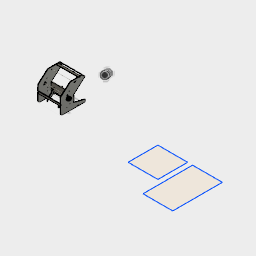
karaoke (Autodesk Fusion 360 design; units mm, degrees)
Autodesk Fusion 360 part; units mm, degrees
(part 1 of 3)
sketch "karaoke_machine_CNC" plane through (0, 0, 0) normal (1, 0, 0) x (0, 0, -1)
  line L0 (-550.0191, 0.004) -> (-575.0344, 25.0175)
  line L1 (-565.5925, 332.4848) -> (-375.0549, 500.0614)
  circle A0 centre (-278.825, 453.825) radius 8.595
  circle A1 centre (-294.0872, 469.0872) radius 1.445
  circle A2 centre (-263.5628, 469.0872) radius 1.445
  circle A3 centre (-294.0872, 438.5628) radius 1.445
  circle A4 centre (-263.5628, 438.5628) radius 1.445
  circle A5 centre (-400, 350) radius 4
  circle A6 centre (-300.125, 453.825) radius 7.88
  circle A7 centre (-380, 180) radius 4
  circle A8 centre (-450, 90) radius 4
  circle A9 centre (-385, 120) radius 4
  circle A10 centre (43.7005, 245.2652) radius 4
  spline S0 degree 5 poles (123.7005, 365.2652) (122.0522, 364.7199) (118.9216, 363.5317) (114.724, 361.457) (110.1257, 358.1046) (106.0037, 352.9433) (103.3614, 346.847) (101.891, 339.898) (101.0418, 332.2492) (100.1108, 324.1052) (98.3724, 315.6927) (95.1998, 307.2345) (90.1793, 298.924) (83.2582, 290.8942) (74.6972, 283.2208) (64.9664, 275.9336) (54.6633, 269.0254) (44.4241, 262.4607) (34.8373, 256.1846) (26.3611, 250.1305) (19.2237, 244.2286) (13.4655, 238.4105) (9.0045, 232.6126) (5.6928, 226.78) (3.3728, 220.8704) (1.9392, 214.8586) (1.457, 209.9581) (1.4586, 206.23) (1.6207, 203.7212) (1.742, 202.461) knots 0 0 0 0 0 0 0.04 0.08 0.12 0.16 0.2 0.24 0.28 0.32 0.36 0.4 0.44 0.48 0.52 0.56 0.6 0.64 0.68 0.72 0.76 0.8 0.84 0.88 0.92 0.96 1 1 1 1 1 1
  line L2 (123.7005, 365.2652) -> (143.7005, 365.2652)
  circle A11 centre (108.7005, 275.2652) radius 4
  circle A12 centre (113.7005, 335.2652) radius 4
  spline S1 degree 5 poles (143.7005, 365.2652) (142.5207, 363.6794) (140.2638, 360.5375) (137.1859, 355.9139) (133.6982, 349.93) (130.3733, 342.6612) (128.0779, 335.363) (126.8118, 327.4866) (126.5171, 318.2243) (126.7275, 307.7361) (126.8179, 296.5667) (126.1032, 285.5142) (123.9849, 275.3406) (120.1067, 266.502) (114.4031, 259.0526) (107.008, 252.8039) (98.2027, 247.4139) (88.3531, 242.4959) (77.8463, 237.7348) (67.0572, 232.924) (56.3415, 227.9315) (46.021, 222.6873) (36.3716, 217.1625) (27.6109, 211.3538) (19.8803, 205.2637) (13.2549, 198.8948) (8.8635, 193.5794) (6.083, 189.4699) (4.4567, 186.6759) (3.7005, 185.2652) knots 0 0 0 0 0 0 0.04 0.08 0.12 0.16 0.2 0.24 0.28 0.32 0.36 0.4 0.44 0.48 0.52 0.56 0.6 0.64 0.68 0.72 0.76 0.8 0.84 0.88 0.92 0.96 1 1 1 1 1 1
  line L3 (131.9605, 355.3516) -> (123.6339, 309.9117)
  line L4 (1.742, 202.461) -> (3.7005, 185.2652)
  circle A13 centre (-26.463, 282.4606) radius 4
  line L5 (53.537, 402.4606) -> (73.537, 402.4606)
  line L6 (-68.4215, 239.6564) -> (-66.463, 222.4606)
  spline S2 degree 5 poles (73.537, 402.4606) (72.3573, 400.8748) (70.1003, 397.7329) (67.0225, 393.1093) (63.5347, 387.1254) (60.2099, 379.8566) (57.9144, 372.5584) (56.6484, 364.682) (56.3536, 355.4197) (56.564, 344.9315) (56.6544, 333.7621) (55.9397, 322.7096) (53.8214, 312.536) (49.9432, 303.6974) (44.2396, 296.248) (36.8445, 289.9993) (28.0392, 284.6094) (18.1896, 279.6913) (7.6828, 274.9302) (-3.1063, 270.1194) (-13.822, 265.127) (-24.1425, 259.8827) (-33.7919, 254.3579) (-42.5526, 248.5492) (-50.2832, 242.4591) (-56.9086, 236.0902) (-61.3, 230.7748) (-64.0805, 226.6653) (-65.7068, 223.8713) (-66.463, 222.4606) knots 0 0 0 0 0 0 0.04 0.08 0.12 0.16 0.2 0.24 0.28 0.32 0.36 0.4 0.44 0.48 0.52 0.56 0.6 0.64 0.68 0.72 0.76 0.8 0.84 0.88 0.92 0.96 1 1 1 1 1 1
  line L7 (61.797, 392.547) -> (53.4704, 347.1071)
  circle A14 centre (38.537, 312.4606) radius 4
  circle A15 centre (43.537, 372.4606) radius 4
  spline S3 degree 5 poles (53.537, 402.4606) (51.8887, 401.9153) (48.7582, 400.7271) (44.5605, 398.6524) (39.9622, 395.3) (35.8403, 390.1387) (33.1979, 384.0424) (31.7275, 377.0934) (30.8784, 369.4446) (29.9473, 361.3006) (28.2089, 352.8881) (25.0363, 344.4299) (20.0159, 336.1194) (13.0947, 328.0896) (4.5337, 320.4162) (-5.1971, 313.129) (-15.5002, 306.2208) (-25.7393, 299.6561) (-35.3261, 293.38) (-43.8023, 287.3259) (-50.9398, 281.424) (-56.698, 275.6059) (-61.159, 269.808) (-64.4707, 263.9754) (-66.7907, 258.0658) (-68.2242, 252.054) (-68.7065, 247.1535) (-68.7049, 243.4254) (-68.5428, 240.9166) (-68.4215, 239.6564) knots 0 0 0 0 0 0 0.04 0.08 0.12 0.16 0.2 0.24 0.28 0.32 0.36 0.4 0.44 0.48 0.52 0.56 0.6 0.64 0.68 0.72 0.76 0.8 0.84 0.88 0.92 0.96 1 1 1 1 1 1
  line L8 (-597.7644, -31.7077) -> (-597.7644, -51.7032)
  line L9 (-597.7763, -161.7146) -> (-597.7763, -141.7146)
  line L10 (-312.3162, 219.9099) -> (-312.3331, 234.9601)
  line L11 (-309.8393, 237.6116) -> (-299.7645, 237.6116)
  line L12 (-299.7645, 217.4116) -> (-309.8145, 217.4116)
  arc A16 (-312.3162, 219.9099) -> (-309.8145, 217.4116) centre (-312.3145, 217.4099) ccw
  arc A17 (-309.8393, 237.6116) -> (-312.3331, 234.9601) centre (-312.3347, 237.4601) ccw
  line L13 (-585.2646, -21.7077) -> (-145.2646, -21.7033)
  line L14 (-585.2759, -171.7145) -> (-145.2759, -171.7005)
  line L15 (-142.8943, -31.6974) -> (-132.8943, -31.6974)
  line L16 (-132.8943, -31.6974) -> (-132.8943, -51.7032)
  line L17 (-132.8943, -51.7032) -> (-142.8887, -51.7032)
  line L18 (-133.0064, -161.6675) -> (-133.0064, -141.7032)
  line L19 (-585.253, -29.2077) -> (-585.2646, -21.7077)
  line L20 (-585.3327, -54.2032) -> (-585.3327, -139.2151)
  line L21 (-585.2785, -164.2145) -> (-585.2759, -171.7145)
  line L22 (-145.3891, -54.197) -> (-145.3747, -139.2034)
  line L23 (-145.2785, -164.1551) -> (-145.2759, -171.7005)
  line L24 (-145.2646, -21.7033) -> (-145.2644, -29.2004)
  arc A18 (-145.3946, -34.197) -> (-142.8943, -31.6974) centre (-145.3943, -31.697) ccw
  arc A19 (-145.2644, -29.2004) -> (-145.3946, -34.197) centre (-145.3943, -31.697) ccw
  arc A20 (-145.3883, -49.197) -> (-145.3891, -54.197) centre (-145.3887, -51.697) ccw
  arc A21 (-142.8887, -51.7032) -> (-145.3883, -49.197) centre (-145.3887, -51.697) ccw
  arc A22 (-145.3747, -139.2034) -> (-145.3328, -144.2032) centre (-145.3328, -141.7031) ccw
  arc A23 (-143.0064, -161.6675) -> (-145.5046, -159.1655) centre (-145.5064, -161.6655) ccw
  arc A24 (-145.5046, -159.1655) -> (-145.2785, -164.1551) centre (-145.5064, -161.6655) ccw
  arc A25 (-587.7774, -141.7146) -> (-585.2773, -144.2145) centre (-585.2774, -141.7145) ccw
  arc A26 (-585.2773, -144.2145) -> (-585.3327, -139.2151) centre (-585.2774, -141.7145) ccw
  arc A27 (-585.2764, -159.2145) -> (-587.7763, -161.7146) centre (-585.2763, -161.7145) ccw
  arc A28 (-585.2785, -164.2145) -> (-585.2764, -159.2145) centre (-585.2763, -161.7145) ccw
  arc A29 (-585.3328, -49.2032) -> (-587.8328, -51.7032) centre (-585.3328, -51.7032) ccw
  arc A30 (-585.3327, -54.2032) -> (-585.3328, -49.2032) centre (-585.3328, -51.7032) ccw
  arc A31 (-587.7644, -31.7077) -> (-585.2643, -34.2077) centre (-585.2644, -31.7077) ccw
  arc A32 (-585.2643, -34.2077) -> (-585.253, -29.2077) centre (-585.2644, -31.7077) ccw
  arc A33 (-145.3328, -144.2032) -> (-142.8328, -141.7032) centre (-145.3328, -141.7032) ccw
  line L25 (-133.0064, -141.7032) -> (-142.8328, -141.7032)
  line L26 (-143.0064, -161.6675) -> (-133.0064, -161.6675)
  line L27 (-587.7644, -31.7077) -> (-597.7644, -31.7077)
  line L28 (-597.7644, -51.7032) -> (-587.8328, -51.7032)
  line L29 (-597.7763, -141.7146) -> (-587.7774, -141.7146)
  line L30 (-587.7763, -161.7146) -> (-597.7763, -161.7146)
  line L31 (-575.4928, 198.8808) -> (-575.7799, 309.8801)
  line L32 (-575.0344, 25.0175) -> (-575.493, 178.6808)
  line L33 (-562.9429, 196.3808) -> (-562.9435, 181.3308)
  line L34 (-565.439, 178.6808) -> (-575.493, 178.6808)
  line L35 (-575.4928, 198.8808) -> (-565.4428, 198.8808)
  arc A34 (-562.9429, 196.3808) -> (-565.4428, 198.8808) centre (-562.9428, 198.8808) ccw
  arc A35 (-565.439, 178.6808) -> (-562.9435, 181.3308) centre (-562.9435, 178.8308) ccw
  arc A36 (-182.4468, 487.9507) -> (-179.7968, 490.4462) centre (-179.9468, 487.9507) ccw
  line L36 (-179.7968, 500.0318) -> (-179.7968, 490.4462)
  line L37 (-182.4468, 487.9507) -> (-197.5, 487.9508)
  line L38 (-199.9968, 490.45) -> (-199.9968, 500.0323)
  arc A37 (-199.9968, 490.45) -> (-197.5, 487.9508) centre (-200, 487.95) ccw
  line L39 (-375.0549, 500.0614) -> (-199.9968, 500.0323)
  line L40 (-179.7968, 500.0318) -> (-124.9386, 500.0255)
  line L41 (-607.4311, 2.1633) -> (-627.4311, 2.1468)
  line L42 (-637.4292, 14.6466) -> (-637.4346, 454.6466)
  line L43 (-597.4308, 454.6468) -> (-597.4308, 14.6571)
  line L44 (-607.4355, 467.1466) -> (-627.4355, 467.1622)
  arc A38 (-627.4313, 12.1468) -> (-629.9313, 14.6468) centre (-627.4313, 14.6468) ccw
  line L45 (-629.9313, 14.6468) -> (-637.4292, 14.6466)
  line L46 (-627.4311, 2.1468) -> (-627.4313, 12.1468)
  line L47 (-607.431, 12.1571) -> (-607.4311, 2.1633)
  line L48 (-597.4308, 14.6571) -> (-604.931, 14.6571)
  line L49 (-637.4346, 454.6466) -> (-629.9354, 454.6466)
  line L50 (-627.4355, 467.1622) -> (-627.4354, 457.1467)
  line L51 (-607.4354, 457.1466) -> (-607.4355, 467.1466)
  line L52 (-604.9354, 454.6467) -> (-597.4308, 454.6468)
  arc A39 (-607.4354, 457.1466) -> (-604.9354, 454.6467) centre (-607.4354, 454.6466) ccw
  arc A40 (-629.9354, 454.6466) -> (-627.4354, 457.1467) centre (-627.4354, 454.6467) ccw
  arc A41 (-604.931, 14.6571) -> (-607.431, 12.1571) centre (-607.431, 14.6571) ccw
  arc A42 (-669.7101, -227.9538) -> (-672.2101, -225.4537) centre (-669.7101, -225.4538) ccw
  line L53 (-229.655, -227.9918) -> (-229.655, -235.4805)
  arc A43 (-227.1554, -225.4914) -> (-229.655, -227.9918) centre (-229.6554, -225.4918) ccw
  arc A44 (-229.6531, -202.9918) -> (-227.1528, -205.4915) centre (-229.6528, -205.4918) ccw
  line L54 (-669.7101, -235.4805) -> (-669.7101, -227.9538)
  line L55 (-227.1554, -225.4914) -> (-217.1554, -225.4914)
  arc A45 (-672.1536, -205.4537) -> (-669.6531, -202.9539) centre (-669.6536, -205.4539) ccw
  line L56 (-229.6531, -195.4805) -> (-229.6531, -202.9918)
  line L57 (-217.1554, -205.4915) -> (-227.1528, -205.4915)
  line L58 (-217.1554, -225.4914) -> (-217.1554, -205.4915)
  line L59 (-682.1536, -225.4537) -> (-682.1536, -205.4537)
  line L60 (-669.6531, -202.9539) -> (-669.6531, -195.4805)
  line L61 (-672.2101, -225.4537) -> (-682.1536, -225.4537)
  line L62 (-682.1536, -205.4537) -> (-672.1536, -205.4537)
  line L63 (-229.655, -235.4805) -> (-669.7101, -235.4805)
  line L64 (-669.6531, -195.4805) -> (-229.6531, -195.4805)
  line L65 (-214.0002, 187.7845) -> (-264.0002, 187.7845)
  line L66 (-269.0002, 194.7845) -> (-264.0002, 187.7845)
  line L67 (-264.0002, 237.7845) -> (-269.0002, 237.7845)
  line L68 (-214.0002, 237.7845) -> (-209.0002, 237.7845)
  line L69 (-264.0002, 242.7845) -> (-264.0002, 249.7845)
  line L70 (-269.0002, 237.7845) -> (-269.0002, 194.7845)
  arc A46 (-264.0002, 237.7845) -> (-264.0002, 242.7845) centre (-264.0002, 240.2845) ccw
  line L71 (-209.0002, 237.7845) -> (-209.0002, 194.7845)
  arc A47 (-214.0002, 242.7845) -> (-214.0002, 237.7845) centre (-214.0002, 240.2845) ccw
  line L72 (-209.0002, 194.7845) -> (-214.0002, 187.7845)
  line L73 (-264.0002, 249.7845) -> (-214.0002, 249.7845)
  line L74 (-214.0002, 249.7845) -> (-214.0002, 242.7845)
  circle A48 centre (-239.0002, 214.7845) radius 4
  line L75 (-173.2818, 321.1956) -> (-130.9318, 321.1956)
  line L76 (-130.9318, 321.1956) -> (-130.9318, 278.8456)
  line L77 (-130.9318, 278.8456) -> (-173.2818, 278.8456)
  line L78 (-173.2818, 278.8456) -> (-173.2818, 321.1956)
  arc A49 (-184.0002, 237.7845) -> (-184.0002, 242.7845) centre (-184.0002, 240.2845) ccw
  line L79 (-184.0002, 242.7845) -> (-184.0002, 249.7845)
  arc A50 (-134.0002, 242.7845) -> (-134.0002, 237.7845) centre (-134.0002, 240.2845) ccw
  line L80 (-129.0002, 237.7845) -> (-129.0002, 194.7845)
  line L81 (-134.0002, 237.7845) -> (-129.0002, 237.7845)
  line L82 (-134.0002, 249.7845) -> (-134.0002, 242.7845)
  line L83 (-189.0002, 194.7845) -> (-184.0002, 187.7845)
  line L84 (-184.0002, 237.7845) -> (-189.0002, 237.7845)
  line L85 (-184.0002, 249.7845) -> (-134.0002, 249.7845)
  line L86 (-134.0002, 187.7845) -> (-184.0002, 187.7845)
  line L87 (-189.0002, 237.7845) -> (-189.0002, 194.7845)
  line L88 (-129.0002, 194.7845) -> (-134.0002, 187.7845)
  line L89 (-173.2818, 206.8396) -> (-173.2818, 208.8983)
  line L90 (-183.2818, 326.1956) -> (-178.2818, 331.1956)
  line L91 (-125.9318, 331.1956) -> (-120.9318, 326.1956)
  line L92 (-183.2818, 273.8456) -> (-178.2818, 268.8456)
  line L93 (-125.9318, 268.8456) -> (-120.9318, 273.8456)
  line L94 (-120.9318, 326.1956) -> (-120.9318, 273.8456)
  line L95 (-183.2818, 273.8456) -> (-183.2818, 326.1956)
  line L96 (-125.9318, 268.8456) -> (-178.2818, 268.8456)
  line L97 (-142.1068, 343.1956) -> (-162.1068, 343.1956)
  arc A51 (-164.6068, 331.1956) -> (-162.1068, 333.6956) centre (-162.1068, 331.1956) ccw
  arc A52 (-142.1068, 333.6956) -> (-139.6068, 331.1956) centre (-142.1068, 331.1956) ccw
  line L98 (-142.1068, 333.6956) -> (-142.1068, 343.1956)
  line L99 (-162.1068, 343.1956) -> (-162.1068, 333.6956)
  line L100 (-178.2818, 331.1956) -> (-164.6068, 331.1956)
  line L101 (-139.6068, 331.1956) -> (-125.9318, 331.1956)
  line L102 (-467, 294.9) -> (-466, 294.9)
  line L103 (-438.025, 304.9) -> (-432.025, 304.9)
  line L104 (-428.025, 300.9) -> (-428.025, 283.9)
  line L105 (-432.025, 279.9) -> (-438.025, 279.9)
  line L106 (-442.025, 283.9) -> (-442.025, 300.9)
  arc A53 (-438.025, 304.9) -> (-442.025, 300.9) centre (-438.025, 300.9) ccw
  arc A54 (-428.025, 300.9) -> (-432.025, 304.9) centre (-432.025, 300.9) ccw
  arc A55 (-432.025, 279.9) -> (-428.025, 283.9) centre (-432.025, 283.9) ccw
  arc A56 (-442.025, 283.9) -> (-438.025, 279.9) centre (-438.025, 283.9) ccw
  circle A57 centre (-447.525, 290.8) radius 4
  line L107 (-460.4181, 236.3812) -> (-460.4102, 228.6812)
  line L108 (-457.9075, 226.1839) -> (-412.7075, 226.234)
  line L109 (-410.2102, 228.7367) -> (-410.2169, 236.3845)
  arc A58 (-410.2169, 236.3845) -> (-412.7175, 238.8839) centre (-410.2175, 238.8845) ccw
  arc A59 (-412.7075, 226.234) -> (-410.2102, 228.7367) centre (-410.2075, 226.2367) ccw
  arc A60 (-457.9209, 238.8839) -> (-460.4181, 236.3812) centre (-460.4209, 238.8812) ccw
  arc A61 (-460.4102, 228.6812) -> (-457.9075, 226.1839) centre (-460.4075, 226.1812) ccw
  line L110 (-412.7175, 238.8839) -> (-457.9209, 238.8839)
  line L111 (-427.3673, 268.2729) -> (-442.5705, 268.286)
  line L112 (-424.8685, 258.0906) -> (-424.8688, 265.7715)
  line L113 (-442.568, 255.586) -> (-427.368, 255.59)
  line L114 (-445.0699, 265.7854) -> (-445.0686, 258.0854)
  arc A62 (-442.5705, 268.286) -> (-445.0699, 265.7854) centre (-445.0705, 268.2854) ccw
  arc A63 (-445.0686, 258.0854) -> (-442.568, 255.586) centre (-445.068, 255.5854) ccw
  arc A64 (-424.8688, 265.7715) -> (-427.3673, 268.2729) centre (-424.8673, 268.2715) ccw
  arc A65 (-427.368, 255.59) -> (-424.8685, 258.0906) centre (-424.868, 255.5906) ccw
  arc A66 (-267.1203, -262.8337) -> (-264.6201, -265.3334) centre (-267.1201, -265.3337) ccw
  line L115 (-254.6212, -265.3334) -> (-264.6201, -265.3334)
  line L116 (-254.6212, -285.3333) -> (-254.6212, -265.3334)
  line L117 (-264.6212, -285.3333) -> (-254.6212, -285.3333)
  arc A67 (-264.6212, -285.3333) -> (-267.1209, -287.8337) centre (-267.1212, -285.3337) ccw
  line L118 (-267.1209, -287.8337) -> (-267.1209, -295.3201)
  line L119 (-267.1209, -295.3201) -> (-707.1787, -295.3201)
  line L120 (-707.1787, -295.3201) -> (-707.1787, -287.7893)
  arc A68 (-707.1787, -287.7893) -> (-709.6786, -285.2892) centre (-707.1786, -285.2893) ccw
  line L121 (-709.6786, -285.2892) -> (-719.6209, -285.2892)
  line L122 (-719.6209, -285.2892) -> (-719.6209, -265.2892)
  line L123 (-719.6209, -265.2892) -> (-709.6209, -265.2892)
  arc A69 (-709.6209, -265.2892) -> (-707.1203, -262.7893) centre (-707.1209, -265.2893) ccw
  line L124 (-707.1203, -262.7893) -> (-707.1203, -255.3201)
  line L125 (-707.1203, -255.3201) -> (-267.1203, -255.3201)
  line L126 (-267.1203, -255.3201) -> (-267.1203, -262.8337)
  arc A70 (-691.1734, 271.1544) -> (-688.6739, 273.6549) centre (-688.6734, 271.1549) ccw
  line L127 (-688.6757, 283.6693) -> (-688.6739, 273.6549)
  line L128 (-668.676, 283.659) -> (-688.6757, 283.6693)
  line L129 (-668.6739, 273.659) -> (-668.676, 283.659)
  arc A71 (-668.6739, 273.659) -> (-666.1734, 271.1595) centre (-668.6734, 271.159) ccw
  line L130 (-666.1734, 271.1595) -> (-658.624, 271.1612)
  line L131 (-658.624, 271.1612) -> (-658.624, -168.7414)
  line L132 (-658.624, -168.7414) -> (-666.0174, -168.7419)
  arc A72 (-666.0174, -168.7419) -> (-668.5172, -171.2422) centre (-668.5174, -168.7422) ccw
  line L133 (-668.5172, -171.2422) -> (-668.5103, -181.3247)
  line L134 (-668.5103, -181.3247) -> (-688.5103, -181.3433)
  line L135 (-688.5103, -181.3433) -> (-688.5208, -171.3433)
  arc A73 (-688.5208, -171.3433) -> (-691.0214, -168.8456) centre (-688.5214, -168.8433) ccw
  line L136 (-691.0214, -168.8456) -> (-698.6005, -168.8472)
  line L137 (-698.6005, -168.8472) -> (-698.6926, 271.1528)
  line L138 (-698.6926, 271.1528) -> (-691.1734, 271.1544)
  line L139 (-124.9386, 500.0255) -> (-115.0588, 490.1431)
  line L140 (-100.7744, 475.8603) -> (-82.3466, 457.4222)
  line L141 (-115.0588, 490.1431) -> (-122.1649, 483.0363)
  line L142 (-107.8637, 468.7638) -> (-100.7744, 475.8603)
  line L143 (-122.1617, 479.5008) -> (-111.3992, 468.7607)
  arc A74 (-111.3992, 468.7607) -> (-107.8637, 468.7638) centre (-109.6299, 466.9945) ccw
  arc A75 (-122.1649, 483.0363) -> (-122.1617, 479.5008) centre (-123.9311, 481.267) ccw
  arc A76 (-227.4836, 12.5647) -> (-229.989, 10.0703) centre (-229.9835, 12.5703) ccw
  arc A77 (-209.789, 10.0247) -> (-212.2834, 12.5304) centre (-209.7834, 12.5247) ccw
  line L144 (-212.2834, 12.5304) -> (-227.4836, 12.5647)
  line L145 (-209.789, 0.0184) -> (-209.789, 10.0247)
  line L146 (-229.989, 10.0703) -> (-229.989, 0.0203)
  line L147 (-74.9996, 0.0054) -> (-209.789, 0.0184)
  line L148 (-229.989, 0.0203) -> (-550.0191, 0.004)
  line L149 (-82.778, 442.8771) -> (-298.0853, 251.6001)
  line L150 (-298.2447, 100.206) -> (-82.7348, 51.894)
  line L151 (-74.9996, 0.0054) -> (-74.9222, 42.1178)
  arc A78 (-82.778, 442.8771) -> (-82.3466, 457.4222) centre (-89.4196, 450.3531) ccw
  arc A79 (-74.9222, 42.1178) -> (-82.7348, 51.894) centre (-84.9222, 42.1362) ccw
  arc A80 (-565.5925, 332.4848) -> (-575.7799, 309.8801) centre (-545.7801, 309.9577) ccw
  line L152 (-299.7645, 247.8621) -> (-299.7645, 237.6116)
  line L153 (-312.3465, 124.9133) -> (-312.305, 109.7134)
  line L154 (-299.798, 127.4147) -> (-309.848, 127.4147)
  line L155 (-309.8037, 107.2147) -> (-299.7978, 107.2147)
  line L156 (-299.7645, 217.4116) -> (-299.798, 127.4147)
  line L157 (-299.7978, 107.2147) -> (-299.8072, 102.1613)
  arc A81 (-309.848, 127.4147) -> (-312.3465, 124.9133) centre (-312.348, 127.4133) ccw
  arc A82 (-312.305, 109.7134) -> (-309.8037, 107.2147) centre (-312.3037, 107.2134) ccw
  arc A83 (-299.8072, 102.1613) -> (-298.2447, 100.206) centre (-297.8072, 102.1576) ccw
  arc A84 (-298.0853, 251.6001) -> (-299.7645, 247.8621) centre (-294.7645, 247.8621) ccw
  line L158 (258.1334, -36.2864) -> (248.0834, -36.2806)
  arc A85 (-234.4099, -279.8571) -> (-234.8601, -294.4016) centre (-227.778, -287.3416) ccw
  circle A86 centre (133.1102, 72.7434) radius 4
  arc A87 (-7.0506, 35.2879) -> (-4.532, 37.7686) centre (-4.5507, 35.2687) ccw
  line L159 (-6.901, 55.5005) -> (-16.9364, 55.5539)
  line L160 (95.6318, -111.3946) -> (140.8389, -111.5507)
  line L161 (93.1338, -101.384) -> (93.1342, -108.8922)
  arc A88 (247.8794, -171.2295) -> (258.125, -148.6539) centre (228.125, -148.6516) ccw
  line L162 (143.3375, -109.0493) -> (143.3342, -101.3493)
  arc A89 (-4.4202, 52.9814) -> (-6.901, 55.5005) centre (-4.4011, 55.4813) ccw
  line L163 (-16.9364, 55.5539) -> (-16.94, 61.1402)
  circle A90 centre (68.1102, 42.7434) radius 4
  line L164 (111.1352, -138.1566) -> (111.1352, -121.1566)
  line L165 (248.3624, -16.0807) -> (258.1446, -16.0865)
  circle A91 centre (63.1102, -17.2566) radius 4
  line L166 (245.5848, -33.7792) -> (245.8652, -18.7291)
  circle A92 centre (130.6352, -128.0566) radius 4
  line L167 (140.8327, -98.8507) -> (95.6327, -98.8828)
  line L168 (233.1135, 162.735) -> (258.1053, 137.7415)
  line L169 (258.1053, 137.7415) -> (258.1446, -16.0865)
  line L170 (258.1334, -36.2864) -> (258.125, -148.6539)
  line L171 (115.1352, -117.1566) -> (121.1352, -117.1566)
  arc A93 (-16.94, 61.1402) -> (-18.5065, 63.0914) centre (-18.94, 61.1389) ccw
  line L172 (-234.4099, -279.8571) -> (-18.696, -88.7172)
  line L173 (150.1102, -132.1566) -> (149.1102, -132.1566)
  line L174 (-16.9682, -54.751) -> (-6.9182, -54.7819)
  arc A94 (-4.4216, -57.2636) -> (-6.9182, -54.7819) centre (-4.4183, -54.7636) ccw
  arc A95 (-204.2696, -307.2898) -> (-207.8051, -307.3083) centre (-206.0466, -305.5313) ccw
  arc A96 (-89.5643, 150.2544) -> (-87.0659, 152.756) centre (-87.0643, 150.256) ccw
  line L175 (-87.0659, 152.756) -> (-87.0759, 162.8059)
  line L176 (-116.8873, -327.7066) -> (-116.8873, -337.2646)
  line L177 (-191.9082, -337.2692) -> (-200.515, -328.6595)
  line L178 (-134.4374, -325.2073) -> (-119.3898, -325.2072)
  line L179 (-107.2759, 162.797) -> (-107.2657, 152.6896)
  line L180 (58.1172, -337.2609) -> (-116.8873, -337.2646)
  line L181 (-137.0873, -337.265) -> (-191.9082, -337.2692)
  line L182 (-200.515, -328.6595) -> (-193.446, -321.5159)
  line L183 (-193.4645, -317.9804) -> (-204.2696, -307.2898)
  line L184 (-214.8733, -314.451) -> (-234.8601, -294.4016)
  line L185 (-207.8051, -307.3083) -> (-214.8733, -314.451)
  arc A97 (-193.446, -321.5159) -> (-193.4645, -317.9804) centre (-191.6875, -319.7388) ccw
  arc A98 (-134.4374, -325.2073) -> (-137.0873, -327.7028) centre (-136.9374, -325.2073) ccw
  arc A99 (-116.8873, -327.7066) -> (-119.3898, -325.2072) centre (-116.8898, -325.2066) ccw
  line L186 (-137.0873, -337.265) -> (-137.0873, -327.7028)
  line L187 (-104.7599, 150.1953) -> (-89.5643, 150.2544)
  line L188 (-16.9682, -54.751) -> (-17.1004, 35.3546)
  line L189 (-87.0759, 162.8059) -> (233.1135, 162.735)
  line L190 (-4.532, 37.7686) -> (-4.4202, 52.9814)
  line L191 (-18.5065, 63.0914) -> (-234.0689, 110.9598)
  line L192 (247.8794, -171.2295) -> (58.1172, -337.2609)
  line L193 (-17.1004, 35.3546) -> (-7.0506, 35.2879)
  line L194 (-241.9076, 162.7375) -> (-241.9011, 120.7205)
  line L195 (-241.9076, 162.7375) -> (-107.2759, 162.797)
  circle A100 centre (-16.7648, -291.0816) radius 7.88
  arc A101 (-18.696, -88.7172) -> (-17.0119, -84.9821) centre (-22.0119, -84.9749) ccw
  arc A102 (125.1352, -121.1566) -> (121.1352, -117.1566) centre (121.1352, -121.1566) ccw
  line L196 (-4.4216, -57.2636) -> (-4.3168, -72.3064)
  arc A103 (248.3624, -16.0807) -> (245.8652, -18.7291) centre (245.8668, -16.2291) ccw
  arc A104 (143.3342, -101.3493) -> (140.8327, -98.8507) centre (143.3327, -98.8493) ccw
  line L197 (-6.7935, -74.9739) -> (-16.9974, -74.951)
  circle A105 centre (83.1102, -187.2566) radius 4
  line L198 (125.1352, -121.1566) -> (125.1352, -138.1566)
  arc A106 (-6.7935, -74.9739) -> (-4.3168, -72.3064) centre (-4.2992, -74.8063) ccw
  arc A107 (140.8389, -111.5507) -> (143.3375, -109.0493) centre (143.3389, -111.5493) ccw
  arc A108 (115.1352, -117.1566) -> (111.1352, -121.1566) centre (115.1352, -121.1566) ccw
  arc A109 (111.1352, -138.1566) -> (115.1352, -142.1566) centre (115.1352, -138.1566) ccw
  line L199 (121.1352, -142.1566) -> (115.1352, -142.1566)
  arc A110 (121.1352, -142.1566) -> (125.1352, -138.1566) centre (121.1352, -138.1566) ccw
  arc A111 (95.6327, -98.8828) -> (93.1338, -101.384) centre (93.1327, -98.884) ccw
  arc A112 (245.5848, -33.7792) -> (248.0834, -36.2806) centre (245.5834, -36.2792) ccw
  line L200 (-17.0119, -84.9821) -> (-16.9974, -74.951)
  arc A113 (93.1342, -108.8922) -> (95.6318, -111.3946) centre (93.1318, -111.3922) ccw
  arc A114 (-241.9011, 120.7205) -> (-234.0689, 110.9598) centre (-231.9011, 120.722) ccw
  arc A115 (-107.2657, 152.6896) -> (-104.7599, 150.1953) centre (-107.2599, 150.1896) ccw
  point P0 (33.7005, 255.2652)
  point P1 (103.242, 345.2652)
  point P2 (93.7005, 305.2652)
  point P3 (5.4606, 225.7294)
  point P4 (131.9605, 355.3516)
  point P5 (123.6339, 309.9117)
  point P6 (124.7708, 280.2227)
  point P7 (93.7005, 245.2652)
  point P8 (33.7005, 215.2652)
  point P9 (127.7972, 332.6316)
  point P10 (23.537, 282.4606)
  point P11 (57.6337, 369.827)
  point P12 (54.6073, 317.4181)
  point P13 (-36.463, 252.4606)
  point P14 (53.4704, 347.1071)
  point P15 (-64.7029, 262.9248)
  point P16 (61.797, 392.547)
  point P17 (33.0785, 382.4606)
  point P18 (23.537, 342.4606)
  point P19 (-36.463, 292.4606)
  point P20 (-442.025, 304.9)
  point P21 (-442.025, 279.9)
  point P22 (125.1352, -142.1566)
  point P23 (125.1352, -117.1566)
  dimension "d40" = 17.19
  dimension "d54" = 2.89
  dimension "d55" = 2.89
  dimension "d56" = 2.89
  dimension "d57" = 2.89
  dimension "d58" = 21.3
  dimension "d60" = 8
  dimension "d86" = 15.76
  dimension "d87" = 8
  dimension "d88" = 8
  dimension "d89" = 8
  dimension "d90" = 8
  dimension "d91" = 8
  dimension "d92" = 8
  dimension "d96" = 8
  dimension "d97" = 8
  dimension "d98" = 8
  dimension "d99" = 12.55
  dimension "d100" = 20.2
  dimension "d103" = 12.5
  dimension "d104" = 20
  dimension "d105" = 12.5
  dimension "d108" = 5
  dimension "d109" = 5
  dimension "d110" = 5
  dimension "d111" = 5
  dimension "d112" = 5
  dimension "d113" = 5
  dimension "d114" = 10
  dimension "d115" = 10
  dimension "d116" = 440
  dimension "d117" = 440
  dimension "d118" = 12.5
  dimension "d119" = 20
  dimension "d121" = 12.5
  dimension "d122" = 5
  dimension "d123" = 5
  dimension "d125" = 5
  dimension "d126" = 20.2
  dimension "d128" = 20.2
  dimension "d129" = 12.55
  dimension "d131" = 5
  dimension "d132" = 5
  dimension "d133" = 5
  dimension "d134" = 12.5
  dimension "d135" = 20
  dimension "d137" = 440
  dimension "d138" = 12.5
  dimension "d139" = 20
  dimension "d140" = 5
  dimension "d141" = 5
  dimension "d142" = 5
  dimension "d143" = 5
  dimension "d144" = 12.5
  dimension "d145" = 20
  dimension "d146" = 440
  dimension "d147" = 12.5
  dimension "d148" = 20
  dimension "d149" = 5
  dimension "d150" = 5
  dimension "d151" = 5
  dimension "d152" = 5
  dimension "d153" = 62
  dimension "d154" = 12
  dimension "d155" = 5
  dimension "d156" = 5
  dimension "d157" = 2.5
  dimension "d158" = 2.5
  dimension "d164" = 8
  dimension "d166" = 42.35
  dimension "d167" = 42.35
  dimension "d170" = 62
  dimension "d171" = 12
  dimension "d172" = 5
  dimension "d173" = 5
  dimension "d174" = 2.5
  dimension "d175" = 2.5
  dimension "d192" = 5
  dimension "d193" = 5
  dimension "d209" = 25
  dimension "d210" = 4
  dimension "d216" = 8
  dimension "d217" = 50.2
  dimension "d218" = 12.7
  dimension "d219" = 5
  dimension "d220" = 5
  dimension "d221" = 5
  dimension "d222" = 5
  dimension "d223" = 12.7
  dimension "d224" = 20.2
  dimension "d225" = 5
  dimension "d226" = 5
  dimension "d227" = 5
  dimension "d228" = 5
  dimension "d229" = 12.5
  dimension "d230" = 20
  dimension "d231" = 440
  dimension "d232" = 12.5
  dimension "d233" = 20
  dimension "d234" = 5
  dimension "d235" = 5
  dimension "d236" = 5
  dimension "d237" = 5
  dimension "d238" = 12.5
  dimension "d239" = 20
  dimension "d240" = 440
  dimension "d241" = 12.5
  dimension "d242" = 20
  dimension "d243" = 5
  dimension "d244" = 5
  dimension "d245" = 5
  dimension "d246" = 5
  dimension "d247" = 12.55
  dimension "d248" = 20.2
  dimension "d249" = 5
  dimension "d250" = 5
  dimension "d251" = 20.2
  dimension "d252" = 12.55
  dimension "d253" = 5
  dimension "d254" = 5
  dimension "d255" = 10
  dimension "d256" = 10
  dimension "d257" = 30
  dimension "d262" = 12.55
  dimension "d263" = 20.2
  dimension "d264" = 5
  dimension "d265" = 5
  dimension "d266" = 2
  dimension "d267" = 5
  dimension "d274" = 8
  dimension "d275" = 15.76
  dimension "d276" = 8
  dimension "d277" = 8
  dimension "d278" = 8
  dimension "d279" = 12.55
  dimension "d280" = 20.2
  dimension "d281" = 5
  dimension "d282" = 5
  dimension "d283" = 20.2
  dimension "d284" = 20.2
  dimension "d285" = 12.55
  dimension "d286" = 5
  dimension "d287" = 5
  dimension "d288" = 5
  dimension "d289" = 25
  dimension "d290" = 4
  dimension "d291" = 8
  dimension "d292" = 50.2
  dimension "d293" = 12.7
  dimension "d294" = 5
  dimension "d295" = 5
  dimension "d296" = 5
  dimension "d297" = 5
  dimension "d304" = 12.55
  dimension "d305" = 20.2
  dimension "d306" = 5
  dimension "d307" = 5
  dimension "d308" = 20.2
  dimension "d309" = 12.55
  dimension "d310" = 5
  dimension "d311" = 5
  dimension "d312" = 10
  dimension "d313" = 10
  dimension "d314" = 30
  dimension "d315" = 12.55
  dimension "d316" = 20.2
  dimension "d317" = 5
  dimension "d318" = 5
  dimension "d319" = 2
  dimension "d320" = 5
  measures "d40" diameter of A0
  measures "d54" diameter of A1
  measures "d55" diameter of A2
  measures "d56" diameter of A3
  measures "d57" diameter of A4
  measures "d58" distance of A0.centre A6.centre
  measures "d60" diameter of A5
  measures "d86" diameter of A6
  measures "d87" diameter of A7
  measures "d88" diameter of A8
  measures "d89" diameter of A9
  measures "d90" diameter of A12
  measures "d91" diameter of A10
  measures "d92" diameter of A11
  measures "d96" diameter of A15
  measures "d97" diameter of A13
  measures "d98" diameter of A14
  measures "d99" distance of L12.start A16.centre
  measures "d100" distance of L12.start L11.end
  measures "d103" distance of L8.start A31.centre
  measures "d104" distance of A25.centre A27.centre
  measures "d105" distance of L9.start A27.centre
  measures "d108" diameter of A17
  measures "d109" diameter of A16
  measures "d110" diameter of A25
  measures "d111" diameter of A29
  measures "d112" diameter of A31
  measures "d113" diameter of A27
  measures "d114" distance of A31.centre L13.start
  measures "d115" distance of A27.centre L14.start
  measures "d116" distance of L13.start L13.end
  measures "d117" distance of L14.start L14.end
  measures "d118" distance of L15.end A18.centre
  measures "d119" distance of A18.centre A20.centre
  measures "d121" distance of L18.start A23.centre
  measures "d122" diameter of A18
  measures "d123" diameter of A20
  measures "d125" diameter of A23
  measures "d126" distance of L38.end L36.start
  measures "d128" distance of L31.start L32.end
  measures "d129" distance of L31.start A34.centre
  measures "d131" diameter of A36
  measures "d132" diameter of A34
  measures "d133" diameter of A35
  measures "d134" distance of L41.end A38.centre
  measures "d135" distance of L41.end L41.start
  measures "d137" distance of L42.start L42.end
  measures "d138" distance of L44.start A39.centre
  measures "d139" distance of A40.centre A39.centre
  measures "d140" diameter of A40
  measures "d141" diameter of A39
  measures "d142" diameter of A38
  measures "d143" diameter of A41
  measures "d144" distance of A45.centre L59.end
  measures "d145" distance of L59.start L59.end
  measures "d146" distance of L56.start L60.end
  measures "d147" distance of L55.end A43.centre
  measures "d148" distance of A44.centre A43.centre
  measures "d149" diameter of A44
  measures "d150" diameter of A43
  measures "d151" diameter of A45
  measures "d152" diameter of A42
  measures "d153" distance of L65.end L69.end
  measures "d154" distance of L69.end L67.start
  measures "d155" distance of L67.end L67.start
  measures "d156" distance of L68.start L68.end
  measures "d157" distance of A46.centre L67.start
  measures "d158" distance of A47.centre L68.start
  measures "d164" diameter of A48
  measures "d166" distance of L75.start L75.end
  measures "d167" distance of L75.start L77.end
  measures "d170" distance of L79.end L83.end
  measures "d171" distance of A49.start L79.end
  measures "d172" distance of A49.start L84.end
  measures "d173" distance of L80.start A50.end
  measures "d174" distance of A49.start A49.centre
  measures "d175" distance of A50.centre A50.end
  measures "d192" diameter of A51
  measures "d193" diameter of A52
  measures "d209" distance of P20 P21
  measures "d210" radius of A53
  measures "d216" diameter of A57
  measures "d217" distance of A61.centre A59.centre
  measures "d218" distance of A60.centre A61.centre
  measures "d219" diameter of A60
  measures "d220" diameter of A61
  measures "d221" diameter of A58
  measures "d222" diameter of A59
  measures "d223" distance of A62.centre A63.centre
  measures "d224" distance of A65.centre A63.centre
  measures "d225" diameter of A62
  measures "d226" diameter of A64
  measures "d227" diameter of A65
  measures "d228" diameter of A63
  measures "d229" distance of A69.centre L122.end
  measures "d230" distance of L121.end L122.end
  measures "d231" distance of L125.end L124.end
  measures "d232" distance of L116.start A67.centre
  measures "d233" distance of A66.centre A67.centre
  measures "d234" diameter of A66
  measures "d235" diameter of A67
  measures "d236" diameter of A69
  measures "d237" diameter of A68
  measures "d238" distance of A73.centre L134.end
  measures "d239" distance of L133.end L134.end
  measures "d240" distance of L137.end L136.end
  measures "d241" distance of L128.start A71.centre
  measures "d242" distance of A70.centre A71.centre
  measures "d243" diameter of A70
  measures "d244" diameter of A71
  measures "d245" diameter of A73
  measures "d246" diameter of A72
  measures "d247" distance of L139.end A75.centre
  measures "d248" distance of L139.end L140.start
  measures "d249" diameter of A75
  measures "d250" diameter of A74
  measures "d251" distance of L146.end L145.start
  measures "d252" distance of L146.end A76.centre
  measures "d253" diameter of A76
  measures "d254" diameter of A77
  measures "d255" radius of A78
  measures "d256" radius of A79
  measures "d257" radius of A80
  measures "d262" distance of L154.start A81.centre
  measures "d263" distance of L154.start L155.end
  measures "d264" diameter of A81
  measures "d265" diameter of A82
  measures "d266" radius of A83
  measures "d267" radius of A84
  measures "d274" diameter of A105
  measures "d275" diameter of A100
  measures "d276" diameter of A91
  measures "d277" diameter of A86
  measures "d278" diameter of A90
  measures "d279" distance of A94.centre L174.start
  measures "d280" distance of L197.end L174.start
  measures "d281" diameter of A106
  measures "d282" diameter of A94
  measures "d283" distance of L176.end L181.start
  measures "d284" distance of L158.start L165.end
  measures "d285" distance of A112.centre L158.start
  measures "d286" diameter of A98
  measures "d287" diameter of A112
  measures "d288" diameter of A103
  measures "d289" distance of P22 P23
  measures "d290" radius of A110
  measures "d291" diameter of A92
  measures "d292" distance of A111.centre A104.centre
  measures "d293" distance of A107.centre A104.centre
  measures "d294" diameter of A107
  measures "d295" diameter of A104
  measures "d296" diameter of A113
  measures "d297" diameter of A111
  measures "d304" distance of L177.end A97.centre
  measures "d305" distance of L177.end L184.start
  measures "d306" diameter of A97
  measures "d307" diameter of A95
  measures "d308" distance of L175.end L179.start
  measures "d309" distance of L175.end A96.centre
  measures "d310" diameter of A96
  measures "d311" diameter of A115
  measures "d312" radius of A85
  measures "d313" radius of A114
  measures "d314" radius of A88
  measures "d315" distance of L188.end A87.centre
  measures "d316" distance of L188.end L159.end
  measures "d317" diameter of A87
  measures "d318" diameter of A89
  measures "d319" radius of A93
  measures "d320" radius of A101